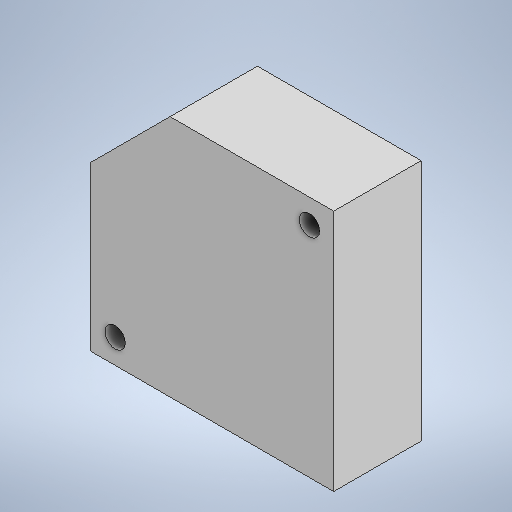
# Autodesk Inventor part: Sensor
Saved by Autodesk Inventor 2025.1 (Build 291241000, 241)
## iProperties
Created: 2025-03-30
Part Number: Sensor
Material: Všeobecné
Document SubType Name: Modeling
Designer: 42060
Density: 1 g/cm^3
Appearance: Výchozí
Author: 42060
Autodesk Inventor part; units mm, degrees
ref_plane "YZ Plane" through (0, 0, 0) normal (1, 0, 0) x (0, 1, 0)
ref_plane "XZ Plane" through (0, 0, 0) normal (0, 1, 0) x (-1, 0, 0)
ref_plane "XY Plane" through (0, 0, 0) normal (0, 0, 1) x (1, 0, 0)
sketch "Náčrt1" plane through (0, 0, 0) normal (0, 0, 1) x (1, 0, 0)
  line L0 (-25, 25) -> (25, 25)
  line L1 (25, 25) -> (25, -25)
  line L2 (25, -25) -> (-25, -25)
  line L3 (-25, -25) -> (-25, 25)
  line L4 (-25, 25) -> (25, -25) construction
  line L5 (25, 25) -> (-25, -25) construction
  line L6 (-25, 8.7) -> (-8.7, 25)
  circle A0 centre (-20, -20) radius 2.1
  circle A1 centre (20, 20) radius 2.1
  point P0 (0, 0)
  dimension "d0" = 50
  dimension "d1" = 50
  dimension "d2" = 33.7
  dimension "d3" = 45
  dimension "d4" = 4.2
  dimension "d6" = 5
  dimension "d7" = 5
  constraints: 14 end point, 4 point on line, 2 centre point, 2 midpoint, 2 parallel, 1 equal radius, 1 horizontal, 1 perpendicular
  measures "d0" distance of L0.end L1.end
  measures "d1" distance of L1.end L2.end
  measures "d2" distance of L0.end L6.end
  measures "d3" angle of L6 L0
  measures "d4" diameter of A1
  measures "d6" distance from line of L0 A1.centre
  measures "d7" distance from line of L2 A0.centre
extrude "Vysunutí1" add sketch "Náčrt1" along normal mid plane 18 contours L0 L1 L2 L3 L6
